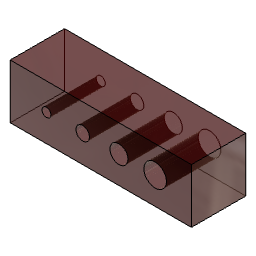
AnyBio_benchmark_negative_features (Autodesk Fusion 360 design; units mm, degrees)
Autodesk Fusion 360 part; units mm, degrees
sketch "Sketch3" plane through (0, 0, 0) normal (0, 0, 1) x (1, 0, 0)
  line L0 (0, 0) -> (10, 0)
  line L1 (10, 0) -> (10, 3)
  line L2 (10, 3) -> (0, 3)
  line L3 (0, 3) -> (0, 0)
  dimension "d15" = 10
  constraint horizontal L0
  constraint vertical L1
  constraint horizontal L2
  constraint vertical L3
  constraint coincident L0.start L3.end
  measures "d15" distance of L0.start L0.end
extrude "Extrude2" add sketch "Sketch3" along normal blind 3
sketch "Sketch4" plane through (0, 0, 0) normal (0, -1, 0) x (1, 0, 0)
  line L0 (0, 0) -> (10, 0)
  line L1 (10, 0) -> (10, 3)
  line L2 (10, 3) -> (0, 3)
  line L3 (0, 3) -> (0, 0)
  line L4 (0, 3) -> (2, 3) construction
  line L5 (2, 3) -> (2, 0) construction
  line L6 (2, 0) -> (0, 0) construction
  line L7 (0, 0) -> (0, 3) construction
  line L8 (2, 3) -> (4, 3) construction
  line L9 (4, 3) -> (4, 0) construction
  line L10 (4, 0) -> (2, 0) construction
  line L11 (2, 0) -> (2, 3) construction
  line L12 (4, 3) -> (6, 3) construction
  line L13 (6, 3) -> (6, 0) construction
  line L14 (6, 0) -> (4, 0) construction
  line L15 (4, 0) -> (4, 3) construction
  line L16 (6, 3) -> (8, 3) construction
  line L17 (8, 3) -> (8, 0) construction
  line L18 (8, 0) -> (6, 0) construction
  line L19 (6, 0) -> (6, 3) construction
  line L20 (0, 1.5) -> (10, 1.5) construction
  circle A0 centre (8, 1.5) radius 0.625
  circle A1 centre (6, 1.5) radius 0.5
  circle A2 centre (4, 1.5) radius 0.375
  circle A3 centre (2, 1.5) radius 0.25
  dimension "d18" = 2
  dimension "d19" = 3
  dimension "d20" = 2
  dimension "d21" = 3
  dimension "d22" = 2
  dimension "d23" = 3
  dimension "d24" = 2
  dimension "d25" = 3
  dimension "d26" = 1.25
  dimension "d27" = 1
  dimension "d28" = 0.75
  dimension "d29" = 0.5
  constraint horizontal L4
  constraint vertical L5
  constraint horizontal L6
  constraint vertical L7
  constraint coincident L2.end L3.start
  constraint horizontal L8
  constraint vertical L9
  constraint horizontal L10
  constraint vertical L11
  constraint horizontal L12
  constraint vertical L13
  constraint horizontal L14
  constraint vertical L15
  constraint horizontal L16
  constraint vertical L17
  constraint horizontal L18
  constraint vertical L19
  constraint midpoint L7 L20.start
  constraint midpoint L1 L20.end
  constraint midpoint L17 A0.centre
  constraint midpoint L13 A1.centre
  constraint midpoint L9 A2.centre
  constraint midpoint L11 A3.centre
  measures "d18" distance of L2.end L4.end
  measures "d19" distance of L2.end L0.start
  measures "d20" distance of L4.end L8.end
  measures "d21" distance of L4.end L5.end
  measures "d22" distance of L8.end L12.end
  measures "d23" distance of L8.end L9.end
  measures "d24" distance of L12.end L16.end
  measures "d25" distance of L12.end L13.end
  measures "d26" diameter of A0
  measures "d27" diameter of A1
  measures "d28" diameter of A2
  measures "d29" diameter of A3
extrude "Extrude3" cut sketch "Sketch4" against normal blind 3 contours A0 | A1 | A2 | A3
